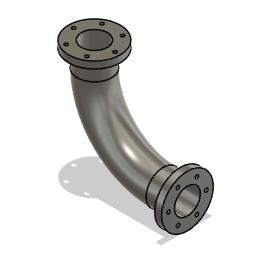
3 v1 (Autodesk Fusion 360 design; units mm, degrees)
Autodesk Fusion 360 part; units mm, degrees
sketch "Sketch1" plane through (0, 0, 0) normal (0, 0, 1) x (1, 0, 0)
  arc A0 (0, 0) -> (200, -200) centre (200, 0) ccw
  dimension "d1" = 400
  constraint coincident origin A0
  measures "d1" diameter of A0
sketch "Sketch2" plane through (0, 0, 0) normal (0, 1, 0) x (1, 0, 0)
  circle A0 centre (0, 0) radius 50
  circle A1 centre (0, 0) radius 37.5
  dimension "d2" = 100
  dimension "d3" = 75
  constraint coincident A0.centre A1.centre
  constraint concentric A0 A1
  measures "d2" diameter of A0
  measures "d3" diameter of A1
sweep "Sweep1" add profiles "Sketch2" path "Sketch1" along A0 section 1 makes body 1
extrude "Extrude1" add 1 faces at (200, -154.3528, 2.484) along direction (1, 0, 0) blind 50 on bodies 1 bodies 1
extrude "Extrude2" add 1 faces at (45.6472, 0, 2.484) along direction (0, 1, 0) blind 50 on bodies 1 bodies 1
sketch "Sketch3" plane through (0, 50, 0) normal (0, 1, 0) x (-1, 0, 0)
  circle A0 centre (0, 0) radius 37.5
  circle A1 centre (0, 0) radius 50
  circle A2 centre (0, 0) radius 75
  dimension "d14" = 150
  constraint concentric A0 A2
  measures "d14" diameter of A2
extrude "Extrude3" add sketch "Sketch3" along normal blind 20 separate body contours A2 makes body 2
sketch "Sketch4" plane through (250, 0, 0) normal (1, 0, 0) x (0, 0, -1)
  circle A0 centre (0, -200) radius 37.5
  circle A1 centre (0, -200) radius 50
  circle A2 centre (0, -200) radius 75
  dimension "d17" = 150
  constraint concentric A0 A2
  measures "d17" diameter of A2
extrude "Extrude4" add sketch "Sketch4" along normal blind 20 separate body contours A2 makes body 3
extrude "Extrude5" add 1 faces at (45.6472, 50, 2.484) along direction (0, 1, 0) blind 20 on bodies 1 bodies 1 2
extrude "Extrude6" add 1 faces at (250, -154.3528, 2.484) along direction (1, 0, 0) blind 20 on bodies 1 bodies 1 3
sketch "Sketch5" plane through (270, 0, 0) normal (1, 0, 0) x (0, 0, -1)
  circle A0 centre (0, -200) radius 37.5
  circle A1 centre (0, -200) radius 75
  circle A2 centre (-55, -200) radius 5
  circle A3 centre (-27.5, -247.6314) radius 5
  circle A4 centre (27.5, -247.6314) radius 5
  circle A5 centre (55, -200) radius 5
  circle A6 centre (27.5, -152.3686) radius 5
  circle A7 centre (-27.5, -152.3686) radius 5
  dimension "d24" = 10
  dimension "d26" = 360
  measures "d24" diameter of A2
extrude "Extrude7" cut sketch "Sketch5" against normal blind 20 contours A2 | A3 | A4 | A5 | A6 | A7 bodies 1
sketch "Sketch6" plane through (0, 70, 0) normal (0, 1, 0) x (-1, 0, 0)
  circle A0 centre (0, 0) radius 37.5
  circle A1 centre (0, 0) radius 75
  circle A2 centre (60, 0) radius 5
  circle A3 centre (30, 51.9615) radius 5
  circle A4 centre (-30, 51.9615) radius 5
  circle A5 centre (-60, 0) radius 5
  circle A6 centre (-30, -51.9615) radius 5
  circle A7 centre (30, -51.9615) radius 5
  dimension "d29" = 10
  dimension "d31" = 360
  measures "d29" diameter of A2
extrude "Extrude8" cut sketch "Sketch6" against normal blind 25 contours A2 | A3 | A4 | A5 | A6 | A7 bodies 1
